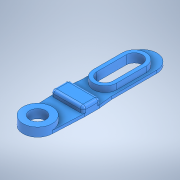
# Autodesk Inventor part: Belt_Restraint
Saved by Autodesk Inventor 2021 (Build 250183000, 183)
## iProperties
Created: 2021-06-13
Part Number: Belt_Restraint
Material: Generic
Document SubType Name: Modeling
Designer: Jorian Brusind
Density: 1 g/cm^3
Appearance: Cyan
Author: Jorian Brusind
Autodesk Inventor part; units mm, degrees
ref_plane "YZ Plane" through (0, 0, 0) normal (1, 0, 0) x (0, 1, 0)
ref_plane "XZ Plane" through (0, 0, 0) normal (0, 1, 0) x (-1, 0, 0)
ref_plane "XY Plane" through (0, 0, 0) normal (0, 0, 1) x (1, 0, 0)
sketch "Sketch15" plane through (0, 0, 0) normal (0, 1, 0) x (-1, 0, 0)
  circle A0 centre (0, 0) radius 2.75
  circle A1 centre (0, 0) radius 5
  line L0 (0, 0) -> (0, -28)
  line L1 (0, -33) -> (0, -23) construction
  line L2 (2.75, -33) -> (2.75, -23)
  line L3 (-2.75, -23) -> (-2.75, -33)
  arc A2 (-2.75, -33) -> (2.75, -33) centre (0, -33) ccw
  arc A3 (2.75, -23) -> (-2.75, -23) centre (0, -23) ccw
  line L4 (0, -43) -> (0, -13) construction
  line L5 (0, 0) -> (0, -14)
  line L6 (-5.5, -15.5) -> (5.5, -15.5)
  line L7 (5.5, -15.5) -> (5.5, -10.5)
  line L8 (5.5, -10.5) -> (-5.5, -10.5)
  line L9 (-5.5, -10.5) -> (-5.5, -15.5)
  line L10 (-5.5, -15.5) -> (5.5, -10.5) construction
  line L11 (5.5, -15.5) -> (-5.5, -10.5) construction
  line L12 (5, 0) -> (5.5, -10.5)
  line L13 (-5, 0) -> (-5.5, -10.5)
  line L14 (0, -35.75) -> (0, -20.25) construction
  line L15 (5, -35.75) -> (5, -20.25)
  line L16 (-5, -20.25) -> (-5, -35.75)
  arc A4 (-5, -35.75) -> (5, -35.75) centre (0, -35.75) ccw
  arc A5 (5, -20.25) -> (-5, -20.25) centre (0, -20.25) ccw
  line L17 (5.5, -15.5) -> (5, -20.25)
  line L18 (-5.5, -15.5) -> (-5, -20.25)
  point P0 (-1.5612, -15.5)
  point P1 (1.5612, -15.5)
  dimension "d102" = 5.5
  dimension "d103" = 10
  dimension "d104" = 28
  dimension "d105" = 5
  dimension "d106" = 5.5
  dimension "d107" = 15
  dimension "d109" = 14
  dimension "d110" = 11
  dimension "d111" = 5
  dimension "d112" = 10
  constraints: 44 end point, 11 point on circle, 8 tangent, 6 centre point, 6 midpoint, 4 parallel, 3 point on line, 2 coincident, 1 horizontal, 1 perpendicular, 1 vertical
  measures "d102" diameter of A0
  measures "d103" diameter of A1
  measures "d104" distance of L0.start L0.end
  measures "d105" distance of L0.end L1.end
  measures "d106" diameter of A3
  measures "d107" distance of L0.end L4.end
  measures "d109" distance of L0.start L5.end
  measures "d110" distance of L8.end L7.end
  measures "d111" distance of L7.end L6.end
  measures "d112" diameter of A5
extrude "Extrusion14" add sketch "Sketch15" along normal blind 1
sketch "Sketch16" plane through (0, 1, 0) normal (0, 1, 0) x (1, 0, 0)
  circle A0 centre (0, 0) radius 2.75 projected
  circle A1 centre (0, 0) radius 2.75
  arc A2 (-5, 0) -> (5, 0) centre (0, 0) ccw projected
  circle A3 centre (0, 0) radius 5
  line L0 (-2.75, 23) -> (-2.75, 33) projected
  line L1 (-2.75, 28) -> (0, 28)
  line L2 (0, 33) -> (0, 23) construction
  line L3 (-2.75, 33) -> (-2.75, 23)
  line L4 (2.75, 23) -> (2.75, 33)
  arc A4 (2.75, 33) -> (-2.75, 33) centre (0, 33) ccw
  arc A5 (-2.75, 23) -> (2.75, 23) centre (0, 23) ccw
  line L5 (0, 33) -> (0, 23) construction
  line L6 (-4, 33) -> (-4, 23)
  line L7 (4, 23) -> (4, 33)
  arc A6 (4, 33) -> (-4, 33) centre (0, 33) ccw
  arc A7 (-4, 23) -> (4, 23) centre (0, 23) ccw
  point P0 (5, 0)
  dimension "d115" = 5
  dimension "d116" = 5.5
  dimension "d117" = 5
  dimension "d118" = 8
  constraints: 18 end point, 8 point on circle, 8 tangent, 5 centre point, 3 equal length, 3 midpoint, 2 coincident, 1 horizontal, 1 vertical, 3 other
  measures "d115" distance of L1.end L2.end
  measures "d116" diameter of A5
  measures "d117" distance of L1.end L2.end
  measures "d118" diameter of A7
extrude "Extrusion15" add sketch "Sketch16" along normal blind 2
sketch "Sketch17" plane through (0, 1, 0) normal (0, 1, 0) x (1, 0, 0)
  line L0 (0, 0) -> (0, 13)
  line L1 (5.5, 16) -> (-5.5, 16)
  line L2 (-5.5, 16) -> (-5.5, 10)
  line L3 (-5.5, 10) -> (5.5, 10)
  line L4 (5.5, 10) -> (5.5, 16)
  line L5 (5.5, 16) -> (-5.5, 10) construction
  line L6 (-5.5, 16) -> (5.5, 10) construction
  dimension "d121" = 13
  dimension "d129" = 11
  dimension "d130" = 6
  constraints: 14 end point, 2 midpoint, 2 parallel, 1 horizontal, 1 perpendicular, 1 vertical
  measures "d121" distance of L0.start L0.end
  measures "d129" distance of L3.end L2.end
  measures "d130" distance of L2.end L1.end
extrude "Extrusion16" add sketch "Sketch17" along normal blind 2
fillet "Fillet7" radius 1 4 edges at (-5.5, 2, -10) (-5.5, 2, -16) (5.5, 2, -10) (5.5, 2, -16)
fillet "Fillet8" radius 1 8 edges at (5.2071, 3, -10.2929) (5.5, 3, -13) (5.2071, 3, -15.7071) (0, 3, -16) (-5.2071, 3, -15.7071) (-5.5, 3, -13) (-5.2071, 3, -10.2929) (0, 3, -10)
body "Solid2"
